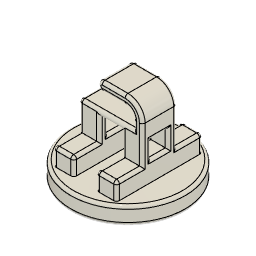
tactorMaking (Autodesk Fusion 360 design; units mm, degrees)
Autodesk Fusion 360 part; units mm, degrees
note: some values were not read from the file. Set by a fixed rule: which sketch regions a step uses.
sketch "Sketch1" plane through (0, 0, 0) normal (0, 1, 0) x (1, 0, 0)
  circle A0 centre (0, 0) radius 10
  dimension "d1" = 20
  constraint coincident A0.centre origin
  measures "d1" diameter of A0
extrude "Extrude1" add sketch "Sketch1" along normal blind 3
fillet "Fillet1" radius 0.5 1 edges at (-9.3233, 3, 3.6162)
fillet "Fillet2" radius 0.5 1 edges at (-9.3233, 0, 3.6162)
sketch "Sketch2" plane through (0, 3, 0) normal (0, 1, 0) x (-1, 0, 0)
  circle A0 centre (0, 0) radius 9.5
  circle A1 centre (0, 0) radius 9.5
  line L0 (2, 7.5) -> (-2, 7.5)
  line L1 (-2, 7.5) -> (-2, -7.5)
  line L2 (-2, -7.5) -> (2, -7.5)
  line L3 (2, -7.5) -> (2, 7.5)
  line L4 (2, 7.5) -> (-2, -7.5) construction
  line L5 (-2, 7.5) -> (2, -7.5) construction
  line L6 (-2, -7.5) -> (-5.5, -7.5)
  line L7 (-5.5, -7.5) -> (-5.5, 7.5)
  line L8 (-5.5, 7.5) -> (-2, 7.5)
  line L9 (-2, 7.5) -> (-2, -7.5)
  line L10 (2, -7.5) -> (5.5, -7.5)
  line L11 (5.5, -7.5) -> (5.5, 7.5)
  line L12 (5.5, 7.5) -> (2, 7.5)
  line L13 (2, 7.5) -> (2, -7.5)
  dimension "d8" = 19
  dimension "d9" = 4
  dimension "d10" = 15
  dimension "d11" = 3.5
  dimension "d12" = 15
  dimension "d13" = 3.5
  dimension "d14" = 15
  constraint concentric A0 A1
  constraint horizontal L0
  constraint perpendicular L0 L1
  constraint parallel L0 L2
  constraint parallel L1 L3
  constraint coincident L4 A0.centre
  constraint coincident L5 A0.centre
  constraint coincident A0.centre A1.centre
  constraint horizontal L6
  constraint vertical L7
  constraint horizontal L8
  constraint vertical L9
  constraint horizontal L10
  constraint vertical L11
  constraint horizontal L12
  constraint vertical L13
  measures "d8" diameter of A1
  measures "d9" distance of L1.end L2.end
  measures "d10" distance of L0.end L1.end
  measures "d11" distance of L1.end L6.end
  measures "d12" distance of L1.end L0.end
  measures "d13" distance of L2.end L10.end
  measures "d14" distance of L2.end L0.start
extrude "Extrude2" add sketch "Sketch2" along normal blind 8 contours L3 L10 L11 L12 L13 | L1 L6 L7 L8 L9
sketch "Sketch3" plane through (5.5, 0, 0) normal (1, 0, 0) x (0, 0, -1)
  line L0 (-7.5, 3) -> (7.5, 3)
  line L1 (7.5, 3) -> (7.5, 11)
  line L2 (7.5, 11) -> (-7.5, 11)
  line L3 (-7.5, 11) -> (-7.5, 3)
  line L4 (0, 3) -> (0, 8) construction
  line L5 (1.5, 9.5) -> (-1.5, 9.5)
  line L6 (-1.5, 9.5) -> (-1.5, 6.5)
  line L7 (-1.5, 6.5) -> (1.5, 6.5)
  line L8 (1.5, 6.5) -> (1.5, 9.5)
  line L9 (1.5, 9.5) -> (-1.5, 6.5) construction
  line L10 (-1.5, 9.5) -> (1.5, 6.5) construction
  point P0 (0, 8)
  dimension "d17" = 5
  dimension "d18" = 3
  dimension "d19" = 3
  constraint midpoint L0 L4.start
  constraint perpendicular L0 L4
  constraint horizontal L5
  constraint perpendicular L5 L6
  constraint parallel L5 L7
  constraint parallel L6 L8
  constraint coincident L9 P0
  constraint coincident L10 P0
  constraint coincident P0 L4.end
  measures "d17" distance of L4.start P0
  measures "d18" distance of L6.end L7.end
  measures "d19" distance of L5.end L6.end
  measures "d38" radius of origin
extrude "Extrude3" cut sketch "Sketch3" against normal blind 16 contours L5 L6 L7 L8
fillet "Fillet3" radius 0.5 16 edges at (5.5, 8, 1.5) (5.5, 9.5, 0) (5.5, 8, -1.5) (5.5, 6.5, 0) (2, 8, 1.5) (2, 9.5, 0) (2, 8, -1.5) (2, 6.5, 0) (-2, 6.5, 0) (-2, 8, 1.5) (-2, 9.5, 0) (-2, 8, -1.5) (-5.5, 8, 1.5) (-5.5, 9.5, 0) (-5.5, 8, -1.5) (-5.5, 6.5, 0)
sketch "Sketch4" plane through (5.5, 0, 0) normal (1, 0, 0) x (0, 0, -1)
  line L0 (-7.5, 3) -> (7.5, 3)
  line L1 (7.5, 3) -> (7.5, 11)
  line L2 (7.5, 11) -> (-7.5, 11)
  line L3 (-7.5, 11) -> (-7.5, 3)
  line L4 (-2, 10) -> (2, 10)
  line L5 (2, 10) -> (2, 6)
  line L6 (2, 6) -> (-2, 6)
  line L7 (-2, 6) -> (-2, 10)
  line L8 (-7.5, 11) -> (-3, 11)
  line L9 (-3, 11) -> (-3, 6)
  line L10 (-3, 6) -> (-7.5, 6)
  line L11 (-7.5, 6) -> (-7.5, 11)
  line L12 (7.5, 11) -> (3, 11)
  line L13 (3, 11) -> (3, 6)
  line L14 (3, 6) -> (7.5, 6)
  line L15 (7.5, 6) -> (7.5, 11)
  dimension "d24" = 4.5
  dimension "d25" = 5
  dimension "d26" = 4.5
  dimension "d27" = 5
  constraint horizontal L8
  constraint vertical L9
  constraint horizontal L10
  constraint vertical L11
  constraint coincident L2.end L3.start
  constraint horizontal L12
  constraint vertical L13
  constraint horizontal L14
  constraint vertical L15
  constraint coincident L1.end L2.start
  measures "d24" distance of L2.end L8.end
  measures "d25" distance of L2.end L10.end
  measures "d26" distance of L1.end L12.end
  measures "d27" distance of L1.end L14.end
extrude "Extrude4" cut sketch "Sketch4" against normal blind 18 contours L2 L3 L8 L9 L10 L11 | L1 L2 L12 L13 L14 L15
sketch "Sketch5" plane through (2, 0, 0) normal (-1, 0, 0) x (0, 0, 1)
  line L0 (-2, 10) -> (2, 10)
  line L1 (2, 10) -> (2, 6)
  line L2 (2, 6) -> (-2, 6)
  line L3 (-2, 6) -> (-2, 10)
  line L4 (7.5, 6) -> (3, 6)
  line L5 (3, 6) -> (3, 11)
  line L6 (3, 11) -> (-3, 11)
  line L7 (-3, 11) -> (-3, 6)
  line L8 (-3, 6) -> (-7.5, 6)
  line L9 (-7.5, 6) -> (-7.5, 3)
  line L10 (-7.5, 3) -> (7.5, 3)
  line L11 (7.5, 3) -> (7.5, 6)
  line L12 (-3, 11) -> (3, 11)
  line L13 (3, 11) -> (3, 10)
  line L14 (3, 10) -> (-3, 10)
  line L15 (-3, 10) -> (-3, 11)
  dimension "d30" = 1
  constraint horizontal L12
  constraint vertical L13
  constraint horizontal L14
  constraint vertical L15
  constraint coincident L6.end L7.start
  measures "d30" distance of L6.end L14.end
extrude "Extrude5" add sketch "Sketch5" along normal blind 4 contours L0 L5 L6 L7 L12 L13 L14 L15
sketch "Sketch6" plane through (0, 0, 3) normal (0, 0, 1) x (1, 0, 0)
  line L0 (2, 10) -> (2, 6)
  line L1 (2, 6) -> (5.5, 6)
  line L2 (5.5, 6) -> (5.5, 11)
  line L3 (5.5, 11) -> (-5.5, 11)
  line L4 (-5.5, 11) -> (-5.5, 6)
  line L5 (-5.5, 6) -> (-2, 6)
  line L6 (-2, 6) -> (-2, 10)
  line L7 (-2, 10) -> (2, 10)
  line L8 (5.5, 11) -> (5.5, 12.5)
  line L9 (2.5, 15.5) -> (-1.5, 15.5)
  line L10 (-1.5, 15.5) -> (-1.5, 14)
  line L11 (-1.5, 14) -> (2.5, 14)
  line L12 (4, 12.5) -> (4, 11)
  arc A0 (5.5, 12.5) -> (2.5, 15.5) centre (2.5, 12.5) ccw
  arc A1 (4, 12.5) -> (2.5, 14) centre (2.5, 12.5) ccw
  circle A2 centre (-1.5, 14.75) radius 0.75
  point P0 (5.5, 15.5)
  point P1 (4, 14)
  dimension "d33" = 4.5
  dimension "d34" = 7
  dimension "d35" = 1.5
  dimension "d36" = 5.5
  dimension "d37" = 3
  dimension "d38" = 1.5
  constraint coincident L2.end L3.start
  constraint perpendicular L3 L8
  constraint perpendicular L8 L9
  constraint perpendicular L9 L10
  constraint perpendicular L10 L11
  constraint coincident L3 L12.end
  constraint perpendicular L3 L12
  constraint coincident P0 L8
  constraint coincident P0 L9
  constraint tangent L8 A0
  constraint tangent L9 A0
  constraint coincident P1 L11
  constraint coincident P1 L12
  constraint tangent L11 A1
  constraint tangent L12 A1
  constraint midpoint L10 A2.centre
  constraint coincident L9.end A2
  measures "d33" distance of L2.end P0
  measures "d34" distance of P0 L9.end
  measures "d35" distance of L9.end L10.end
  measures "d36" distance of L10.end P1
  measures "d37" radius of A0
  measures "d38" radius of A1
extrude "Extrude6" add sketch "Sketch6" against normal blind 6 contours L3 L8 L9 L11 L12 A0 A1 A2 | L10 A2 | L10 A2
fillet "Fillet4" radius 0.5 45 edges at (5.5, 9.25, 3) (4.6213, 14.6213, 3) (0.5, 15.5, 3) (-2.25, 14.75, 3) (0.5, 14, 3) (3.5607, 13.5607, 3) (4, 11.75, 3) (-0.75, 11, 3) (-5.5, 8.5, 3) (-2, 8, 3) (0, 10, 3) (2, 8, 3) (2, 6, 5.25) (5.5, 6, 5.25) (-2, 6, 5.25) (-5.5, 6, 5.25) (-3.75, 6, 7.5) (-5.5, 4.5, 7.5) (-2, 4.5, 7.5) (5.5, 4.5, 7.5) (2, 4.5, 7.5) (3.75, 6, 7.5) (4, 11.75, -3) (3.5607, 13.5607, -3) (0.5, 14, -3) (-2.25, 14.75, -3) (0.5, 15.5, -3) (4.6213, 14.6213, -3) (5.5, 9.25, -3) (-0.75, 11, -3) (-5.5, 11, 0) (-5.5, 8.5, -3) (-5.5, 6, -5.25) (-5.5, 4.5, -7.5) (-2, 8, -3) (0, 10, -3) (2, 8, -3) (2, 6, -5.25) (-2, 6, -5.25) (-2, 4.5, -7.5) (2, 4.5, -7.5) (3.75, 6, -7.5) (-3.75, 6, -7.5) (5.5, 6, -5.25) (5.5, 4.5, -7.5)
